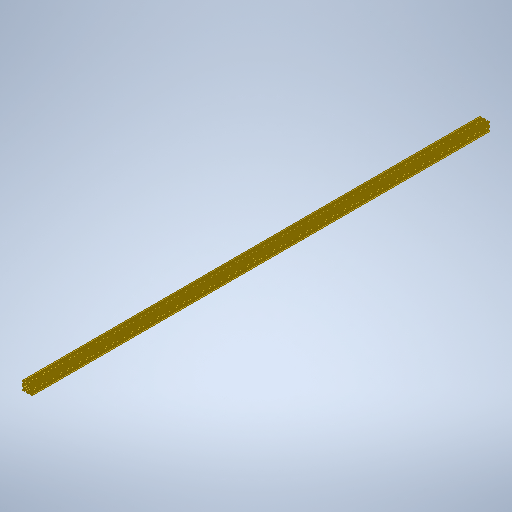
# Autodesk Inventor part: Perfil 40×40 8 rasgos_AST04004008
Saved by Autodesk Inventor 2025.2 (Build 292293000, 293)
## iProperties
Created: 2025-04-03
Part Number: Perfil 40×40 8 rasgos_AST04004008
Material: Ouro
Document SubType Name: Modeling
Designer: Gustavo Sousa
Density: 19.3 g/cm^3
Appearance: Metal quente 2400F
Author: Gustavo Sousa
Autodesk Inventor part; units mm, degrees
ref_plane "YZ Plane" through (0, 0, 0) normal (1, 0, 0) x (0, 1, 0)
ref_plane "XZ Plane" through (0, 0, 0) normal (0, 1, 0) x (-1, 0, 0)
ref_plane "XY Plane" through (0, 0, 0) normal (0, 0, 1) x (1, 0, 0)
sketch "Esboço1" plane through (0, 0, 0) normal (0, 0, 1) x (1, 0, 0)
  line L0 (-20, 20) -> (20, 20) construction
  line L1 (-20, 20) -> (-20, -20) construction
  line L2 (-14, 13.1) -> (-14, 6.9) construction
  line L3 (-20, 20) -> (-20, 0) construction
  line L4 (-20, 13.1) -> (-20, 6.9) construction
  line L5 (-20, 20) -> (-20, 13.1) construction
  line L6 (-20, 13.1) -> (-18, 13.1) construction
  line L7 (-18, 13.1) -> (-18, 17.1) construction
  circle A0 centre (-10, 10) radius 2.5 construction
  line L8 (-10, 10) -> (-20, 20) construction
  line L9 (-18, 17.1) -> (-14, 13.1) construction
  line L10 (-13.1, 14) -> (-6.9, 14) construction
  line L11 (-13.1, 20) -> (-6.9, 20) construction
  line L12 (-20, 20) -> (0, 20) construction
  line L13 (-20, 20) -> (-13.1, 20) construction
  line L14 (-13.1, 20) -> (-13.1, 18) construction
  line L15 (-13.1, 18) -> (-17.1, 18) construction
  line L16 (-17.1, 18) -> (-13.1, 14) construction
  line L17 (-6.9, 20) -> (0, 20) construction
  line L18 (-10, 10) -> (0, 20) construction
  line L19 (-6.9, 20) -> (-6.9, 18) construction
  line L20 (-6.9, 18) -> (-2.9, 18) construction
  line L21 (-2.9, 18) -> (-6.9, 14) construction
  arc A1 (-15.8929, 18) -> (-16.2464, 17.1464) centre (-15.8929, 17.5) ccw
  arc A2 (-13.2464, 14.1464) -> (-12.8929, 14) centre (-12.8929, 14.5) ccw
  arc A3 (-3.7536, 17.1464) -> (-4.1071, 18) centre (-4.1071, 17.5) ccw
  arc A4 (-7.1071, 14) -> (-6.7536, 14.1464) centre (-7.1071, 14.5) ccw
  arc A5 (-19.5, 20) -> (-20, 19.5) centre (-19.5, 19.5) ccw
  line L22 (-13.1, 20) -> (-13.6, 20) construction
  line L23 (-13.6, 20) -> (-13.6, 19.5)
  line L24 (-13.6, 19.5) -> (-13.1, 19.5)
  line L25 (-13.1, 19.5) -> (-13.1, 20) construction
  line L26 (-6.9, 20) -> (-6.4, 20) construction
  line L27 (-6.4, 20) -> (-6.4, 19.5)
  line L28 (-6.4, 19.5) -> (-6.9, 19.5)
  line L29 (-6.9, 19.5) -> (-6.9, 20) construction
  line L30 (-19.5, 20) -> (-13.6, 20)
  line L31 (-13.1, 19.5) -> (-13.1, 18)
  line L32 (-13.1, 18) -> (-15.8929, 18)
  line L33 (-16.2464, 17.1464) -> (-13.2464, 14.1464)
  line L34 (-12.8929, 14) -> (-10, 14)
  line L35 (-10, 14) -> (-7.1071, 14)
  line L36 (-6.7536, 14.1464) -> (-3.7536, 17.1464)
  line L37 (-4.1071, 18) -> (-6.9, 18)
  line L38 (-6.9, 18) -> (-6.9, 19.5)
  line L39 (-6.4, 20) -> (0, 20)
  arc A6 (-14, 12.8929) -> (-14.1464, 13.2464) centre (-14.5, 12.8929) ccw
  arc A7 (-17.1464, 16.2464) -> (-18, 15.8929) centre (-17.5, 15.8929) ccw
  line L40 (-20, 13.1) -> (-19.5, 13.1) construction
  line L41 (-19.5, 13.1) -> (-19.5, 13.6)
  line L42 (-19.5, 13.6) -> (-20, 13.6)
  line L43 (-20, 13.6) -> (-20, 13.1) construction
  line L44 (-20, 19.5) -> (-20, 13.6)
  line L45 (-19.5, 13.1) -> (-18, 13.1)
  line L46 (-18, 13.1) -> (-18, 15.8929)
  line L47 (-17.1464, 16.2464) -> (-14.1464, 13.2464)
  line L48 (-20, 0) -> (-20, 6.9) construction
  line L49 (-20, 6.9) -> (-18, 6.9) construction
  line L50 (-18, 6.9) -> (-18, 2.9) construction
  line L51 (-10, 10) -> (-20, 0) construction
  line L52 (-14, 6.9) -> (-18, 2.9) construction
  arc A8 (-14.1464, 6.7536) -> (-14, 7.1071) centre (-14.5, 7.1071) ccw
  arc A9 (-18, 4.1071) -> (-17.1464, 3.7536) centre (-17.5, 4.1071) ccw
  line L53 (-20, 6.9) -> (-19.5, 6.9) construction
  line L54 (-19.5, 6.9) -> (-19.5, 6.4)
  line L55 (-19.5, 6.4) -> (-20, 6.4)
  line L56 (-20, 6.4) -> (-20, 6.9) construction
  line L57 (-20, 6.4) -> (-20, 0)
  line L58 (-19.5, 6.9) -> (-18, 6.9)
  line L59 (-18, 6.9) -> (-18, 4.1071)
  line L60 (-17.1464, 3.7536) -> (-14.1464, 6.7536)
  line L61 (-14, 7.1071) -> (-14, 10)
  line L62 (-14, 10) -> (-14, 12.8929)
  line L63 (-13.1, 5.9182) -> (-6.9, 5.9182) construction
  line L64 (-20, 0) -> (-19, 0)
  line L65 (-13.1, 5.9182) -> (-18.9294, 0.0889)
  arc A10 (-18.9294, 0.0889) -> (-19, 0) centre (-18.5758, -0.2647) ccw
  line L66 (-13.1, 5.9182) -> (-10, 5.9182)
  arc A11 (-10, 5.9182) -> (-10, 7.5) centre (-10.612, 6.7091) ccw
  arc A12 (-10, 12.5) -> (-12.5, 10) centre (-10, 10) ccw
  arc A13 (-7.5, 10) -> (-10, 12.5) centre (-10, 10) ccw
  arc A14 (-12.5, 10) -> (-10, 7.5) centre (-10, 10) ccw
  line L67 (-5.9159, 13.1) -> (-5.9159, 6.9) construction
  line L68 (0, 20) -> (0, 19)
  line L69 (-5.9159, 13.1) -> (-0.0826, 18.9333) construction
  arc A15 (0, 19) -> (-0.0826, 18.9333) centre (0.2709, 18.5798) ccw
  arc A16 (-7.5, 10) -> (-5.9159, 10) centre (-6.708, 10.6105) ccw
  line L70 (-5.9159, 10) -> (-5.9159, 13.1) construction
  arc A17 (-5.7695, 13.2464) -> (-5.9159, 12.8929) centre (-5.4159, 12.8929) ccw
  line L71 (-5.9159, 12.8929) -> (-5.9159, 10)
  line L72 (-5.7695, 13.2464) -> (-0.0826, 18.9333)
  point P0 (0, 0)
  point P1 (-20, 10)
  point P2 (-20, 10)
  point P3 (-10, 20)
  point P4 (-10, 20)
  point P5 (-19, 6.9)
  point P6 (-6.9, 19)
  dimension "d1" = 40
  dimension "d2" = 20
  dimension "d3" = 6.2
  dimension "d4" = 20
  dimension "d5" = 6
  dimension "d7" = 2
  dimension "d9" = 5
  dimension "d10" = 10
  dimension "d14" = 6
  dimension "d15" = 0.5
  dimension "d16" = 0.5
  dimension "d19" = 4
  dimension "d20" = 0.6942
  dimension "d21" = 1
  dimension "d24" = 0.6958
  constraints: 146 end point, 38 point on circle, 23 collinear, 23 tangent, 20 point on line, 19 equal length, 18 centre point, 14 parallel, 12 equal radius, 11 horizontal, 11 midpoint, 10 vertical, 8 vertical alignment, 6 coincident, 6 perpendicular, 5 horizontal alignment
  measures "d1" distance of L0.start L0.end
  measures "d2" distance from line of point (0, 0) L0
  measures "d3" distance of L2.start L2.end
  measures "d4" distance of L0.start L3.end
  measures "d5" distance between parallel lines of L3 L2
  measures "d7" distance between parallel lines of L1 L7
  measures "d9" diameter of A0
  measures "d10" horizontal distance of point (0, 0) L8.start
  measures "d14" distance between parallel lines of L12 L10
  measures "d15" radius of A5
  measures "d16" distance of L24.end L23.end
  measures "d19" distance from line of L8.start L2
  measures "d20" distance between parallel lines of L51 L65
  measures "d21" radius of A11
  measures "d24" distance between parallel lines of L18 L69
extrude "Extrusão1" add sketch "Esboço1" along normal mid plane 2000
mirror "Espelhar1" about plane through (0, 0, 0) normal (1, 0, 0) of "Extrusão1"
mirror "Espelhar2" about plane through (0, 0, 0) normal (0, 1, 0) of "Extrusão1", "Espelhar1"
fillet "Arredondamento1" radius 1 4 edges at (-19, 0, 0) (19, 0, 0) (0, 19, 0) (0, -19, 0)
